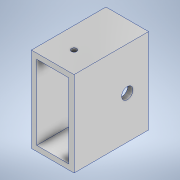
# Autodesk Inventor part: bumper beam
Saved by Autodesk Inventor 2022 (Build 260153000, 153)
## iProperties
Created: 2023-01-12
Part Number: bumper beam
Material: Aluminum 6061
Document SubType Name: Modeling
Designer: S135320
Density: 2.7 g/cm^3
Appearance: Aluminum - Flat
Mass: 75.2958 g
Surface Area: 186.52 cm^2
Volume: 27.8873 cm^3
Author: S135320
Autodesk Inventor part; units mm, degrees
ref_plane "YZ Plane" through (0, 0, 0) normal (1, 0, 0) x (0, 1, 0)
ref_plane "XZ Plane" through (0, 0, 0) normal (0, 1, 0) x (-1, 0, 0)
ref_plane "XY Plane" through (0, 0, 0) normal (0, 0, 1) x (1, 0, 0)
sketch "Sketch1" plane through (0, 0, 0) normal (0, 0, 1) x (1, 0, 0)
  line L0 (0, 0) -> (25.4, 0)
  line L1 (25.4, 0) -> (25.4, 50.8)
  line L2 (25.4, 50.8) -> (0, 50.8)
  line L3 (0, 50.8) -> (0, 0)
  dimension "d0" = 25.4
  dimension "d1" = 50.8
  constraints: 8 end point, 2 parallel, 1 horizontal, 1 perpendicular
  measures "d0" distance of L2.end L1.end
  measures "d1" distance of L1.end L0.end
extrude "Extrusion1" add sketch "Sketch1" along normal blind 44.45
shell "Shell2" thickness 3.175 removed faces 2 at (8.4667, 16.9333, 0) at (8.4667, 16.9333, 44.45)
sketch "Sketch2" plane through (25.4, 0, 0) normal (1, 0, 0) x (0, 0, -1)
  circle A0 centre (-12.7, 25.4) radius 3.3782
  line L0 (0, 0) -> (0, 50.8) projected
  line L1 (0, 50.8) -> (-44.45, 50.8) projected
  dimension "d6" = 12.7
  dimension "d7" = 6.7564
  dimension "d8" = 25.4
  constraints: 1 centre point
  measures "d6" distance from line of L0 A0.centre
  measures "d7" diameter of A0
  measures "d8" distance from line of L1 A0.centre
extrude "Extrusion2" cut sketch "Sketch2" against normal blind 63.5
sketch "Sketch3" plane through (0, 50.8, 0) normal (0, 1, 0) x (1, 0, 0)
  line L0 (25.4, -44.45) -> (0, -44.45) projected
  line L1 (12.7, -44.45) -> (12.7, -31.75)
  circle A0 centre (12.7, -31.75) radius 1.5875
  point P0 (0, 0)
  dimension "d11" = 12.7
  dimension "d12" = 3.175
  constraints: 2 end point, 1 centre point, 1 coincident, 1 midpoint, 1 vertical
  measures "d11" distance of L1.start L1.end
  measures "d12" diameter of A0
extrude "Extrusion3" cut sketch "Sketch3" against normal blind 63.5
body "Solid1"
